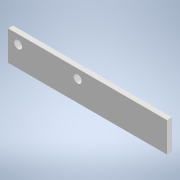
# Autodesk Inventor part: sujetador_motor
Saved by Autodesk Inventor 2022 (Build 260153000, 153)
## iProperties
Created: 2022-03-16
Part Number: sujetador_motor
Material: Generic
Document SubType Name: Modeling
Designer: katha
Density: 1 g/cm^3
Appearance: Default
Author: katha
Autodesk Inventor part; units mm, degrees
ref_plane "YZ Plane" through (0, 0, 0) normal (1, 0, 0) x (0, 1, 0)
ref_plane "XZ Plane" through (0, 0, 0) normal (0, 1, 0) x (-1, 0, 0)
ref_plane "XY Plane" through (0, 0, 0) normal (0, 0, 1) x (1, 0, 0)
sketch "Sketch1" plane through (0, 0, 0) normal (0, 0, 1) x (1, 0, 0)
  circle A0 centre (-173.3589, -112.9) radius 2 projected
  circle A1 centre (-143.3589, -112.9) radius 2 projected
  circle A2 centre (-173.3589, -112.9) radius 2
  circle A3 centre (-143.3589, -112.9) radius 2
  line L0 (-178.3589, -108.4) -> (-98.3589, -108.4)
  line L1 (-98.3589, -108.4) -> (-98.3589, -123.4)
  line L2 (-98.3589, -123.4) -> (-178.3589, -123.4)
  line L3 (-178.3589, -123.4) -> (-178.3589, -108.4)
  point P0 (0, 0)
  dimension "d0" = 4
  dimension "d1" = 4
  dimension "d2" = 15
  dimension "d3" = 80
  dimension "d4" = 4.5
  dimension "d5" = 5
  constraints: 8 end point, 2 centre point, 2 coincident, 2 parallel, 1 horizontal, 1 perpendicular
  measures "d0" diameter of A2
  measures "d1" diameter of A3
  measures "d2" distance between parallel lines of L2 L0
  measures "d3" distance between parallel lines of L1 L3
  measures "d4" distance from line of L0 A0.centre
  measures "d5" distance from line of L3 A0.centre
extrude "Extrusion1" add sketch "Sketch1" along normal blind 2.5
body "Solid1"
